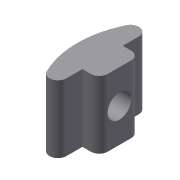
# Autodesk Inventor part: 00_Aluminiumrail_nutslider_block
Saved by Autodesk Inventor 2019.4 (Build 234330000, 330)
## iProperties
Created: 2021-09-23
Part Number: 00_Aluminiumrail_nutslider_block
Material: Generic
Document SubType Name: Modeling
Designer: diederichbenedict
Density: 1 g/cm^3
Appearance: Default
Author: diederichbenedict
Autodesk Inventor part; units mm, degrees
ref_plane "YZ Plane" through (0, 0, 0) normal (1, 0, 0) x (0, 1, 0)
ref_plane "XZ Plane" through (0, 0, 0) normal (0, 1, 0) x (-1, 0, 0)
ref_plane "XY Plane" through (0, 0, 0) normal (0, 0, 1) x (1, 0, 0)
sketch "Sketch1" plane through (0, 0, 0) normal (0, 1, 0) x (-1, 0, 0)
  line L0 (0, 0) -> (0, -2.4)
  line L1 (0, -2.4) -> (2, -2.4)
  line L2 (2, -2.4) -> (2, -6.9)
  line L3 (2, -6.9) -> (2.5, -6.9)
  arc A0 (2.5, -6.9) -> (5, 0) centre (-5.772, 0) ccw
  line L4 (0, 0) -> (5, 0)
  dimension "d0" = 2.4
  dimension "d1" = 2
  dimension "d2" = 4.5
  dimension "d3" = 0.5
  dimension "d14" = 3
  constraints: 10 end point, 3 perpendicular, 2 point on circle, 1 centre point, 1 horizontal, 1 line through centre, 1 vertical
  measures "d0" distance of L0.start L0.end
  measures "d1" distance of L0.end L1.end
  measures "d2" distance of L1.end L2.end
  measures "d3" distance of L2.end L3.end
  measures "d14" horizontal distance of L1.end L4.end
extrude "Extrusion1" add sketch "Sketch1" along normal blind 8
mirror "Mirror1" about plane through (-5, 0, 0) normal (0, 0, 1) of "Extrusion1"
fillet "Fillet1" radius 1 6 edges at (-2, 4, 6.9) (-2.5, 4, 6.9) (-2, 4, -6.9) (-2.5, 4, -6.9) (0, 4, -2.4) (0, 4, 2.4)
sketch "Sketch2" plane through (0, 0, 1.4) normal (1, 0, 0) x (0, 0, -1)
  line L0 (0, 0) -> (0, 8) projected
  line L1 (0, 0) -> (2.8, 0) projected
  line L2 (2.8, 8) -> (2.8, 0) projected
  line L3 (2.8, 8) -> (0, 8) projected
  circle A0 centre (1.4, 4) radius 1.4
  point P0 (1.4, 0)
  dimension "d7" = 2.8
  constraints: 1 centre point
  measures "d7" diameter of A0
extrude "Extrusion2" cut sketch "Sketch2" against normal blind 8 contours A0
ref_plane "Work Plane1" through (-7, 0, 1.4) normal (1, 0, 0) x (0, 0, -1)
sketch "Sketch3" plane through (-7, 0, 1.4) normal (1, 0, 0) x (0, 0, -1)
  line L0 (2.7812, 6.4356) -> (4.1999, 4.0217)
  line L1 (4.1999, 4.0217) -> (2.8187, 1.586)
  line L2 (2.8187, 1.586) -> (0.0188, 1.5644)
  line L3 (0.0188, 1.5644) -> (-1.3999, 3.9783)
  line L4 (-1.3999, 3.9783) -> (-0.0187, 6.414)
  line L5 (-0.0187, 6.414) -> (2.7812, 6.4356)
  line L6 (29.5051, 26.3613) -> (-4.2936, 26.3613) projected
  line L7 (2.8, 8) -> (0, 8) projected
  circle A0 centre (1.4, 4) radius 2.4249 construction
  arc A1 (0, 4) -> (2.8, 4) centre (1.4, 4) ccw construction
  arc A2 (2.8, 4) -> (0, 4) centre (1.4, 4) ccw construction
  line L8 (-2.064, 3.9732) -> (-0.3088, 0.9867)
  line L9 (-0.3088, 0.9867) -> (3.1552, 1.0135)
  line L10 (3.1552, 1.0135) -> (4.864, 4.0268)
  line L11 (4.864, 4.0268) -> (3.1088, 7.0133)
  line L12 (3.1088, 7.0133) -> (-0.3552, 6.9865)
  line L13 (-0.3552, 6.9865) -> (-2.064, 3.9732)
  point P0 (1.4, 0)
  dimension "d11" = 6
  constraints: 24 end point, 3 tangent, 1 centre point, 1 concentric, 1 equal length, 20 other
  measures "d11" distance between parallel lines of L11 L8
extrude "Extrusion3" cut sketch "Sketch3" along normal blind 3 contours L0 L1 L2 L3 L4 L5 | L13 L12 L11 L10 L9 L8
body "Solid1"
